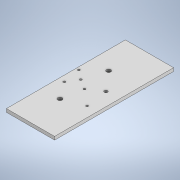
# Autodesk Inventor part: Część1
Saved by Autodesk Inventor 2020 (Build 240168000, 168)
## iProperties
Created: 2019-04-24
Part Number: Część1
Material: Ogólny
Document SubType Name: Modeling
Designer: atmat
Density: 1 g/cm^3
Appearance: Domyślna
Author: atmat
Autodesk Inventor part; units mm, degrees
ref_plane "YZ Plane" through (0, 0, 0) normal (1, 0, 0) x (0, 1, 0)
ref_plane "XZ Plane" through (0, 0, 0) normal (0, 1, 0) x (-1, 0, 0)
ref_plane "XY Plane" through (0, 0, 0) normal (0, 0, 1) x (1, 0, 0)
sketch "Szkic1" plane through (0, 0, 0) normal (0, 1, 0) x (-1, 0, 0)
  circle A0 centre (0, 22.5) radius 2
  circle A1 centre (0, -22.5) radius 2
  circle A2 centre (0, 22.5) radius 11.25 construction
  circle A3 centre (0, -22.5) radius 11.25 construction
  circle A4 centre (0, 0) radius 11.25
  circle A5 centre (-15.3043, -4.6667) radius 4.75 construction
  circle A6 centre (-15.3043, -4.6667) radius 12.25 construction
  circle A7 centre (-18.2464, 15.6211) radius 8.25 construction
  circle A8 centre (-18.2464, 15.6211) radius 1
  circle A9 centre (-15.3043, -4.6667) radius 1.5
  line L0 (17, 55) -> (-27.5543, 55)
  line L1 (-27.5543, 55) -> (-27.5543, -55)
  line L2 (-27.5543, -55) -> (17, -55)
  line L3 (17, -55) -> (17, 55)
  circle A10 centre (0, 22.5) radius 17 construction
  circle A11 centre (0, -22.5) radius 17 construction
  circle A12 centre (0, 0) radius 14.5 construction
  line L4 (12.5, 7.3485) -> (12.5, -7.3485) construction
  line L5 (-12.5, 7.3485) -> (-12.5, -7.3485) construction
  circle A13 centre (14.4557, -9.4125) radius 8.25 construction
  circle A14 centre (14.4557, -9.4125) radius 2.75 construction
  circle A15 centre (11.623, 6.8425) radius 8.25 construction
  circle A16 centre (11.623, 6.8425) radius 1
  circle A17 centre (14.4557, -9.4125) radius 1
  circle A18 centre (5.8715, -2.5341) radius 8.25 construction
  circle A19 centre (5.8715, -2.5341) radius 1
  circle A20 centre (5.8715, -2.5341) radius 2.75 construction
  circle A21 centre (-3.4492, 3.3075) radius 8.25 construction
  circle A22 centre (-3.4492, 3.3075) radius 1
  circle A23 centre (-3.4492, 3.3075) radius 2.75 construction
  dimension "d0" = 4
  dimension "d1" = 4
  dimension "d2" = 22.5
  dimension "d3" = 22.5
  dimension "d4" = 22.5
  dimension "d5" = 22.5
  dimension "d6" = 22.5
  dimension "d7" = 9.5
  dimension "d8" = 24.5
  dimension "d9" = 16.5
  dimension "d10" = 2
  dimension "d11" = 3
  dimension "d12" = 34
  dimension "d13" = 34
  dimension "d14" = 29
  dimension "d15" = 25
  dimension "d16" = 17
  dimension "d17" = 55
  dimension "d18" = 110
  dimension "d21" = 16.5
  dimension "d22" = 5.5
  dimension "d23" = 16.5
  dimension "d24" = 45
  dimension "d26" = 2
  dimension "d27" = 2
  dimension "d28" = 16.5
  dimension "d29" = 2
  dimension "d30" = 5.5
  dimension "d33" = 16.5
  dimension "d34" = 27.5543
  dimension "d35" = 2
  dimension "d36" = 5.5
  constraints: 24 centre point, 16 coincident, 13 tangent, 12 end point, 4 parallel, 4 point on circle, 1 horizontal, 1 perpendicular, 1 vertical
  measures "d0" diameter of A0
  measures "d1" diameter of A1
  measures "d2" distance of point (0, 0) A0.centre
  measures "d3" distance of point (0, 0) A1.centre
  measures "d4" diameter of A2
  measures "d5" diameter of A3
  measures "d6" diameter of A4
  measures "d7" diameter of A5
  measures "d8" diameter of A6
  measures "d9" diameter of A7
  measures "d10" diameter of A8
  measures "d11" diameter of A9
  measures "d12" diameter of A10
  measures "d13" diameter of A11
  measures "d14" diameter of A12
  measures "d15" distance between parallel lines of L4 L5
  measures "d16" distance from line of L3 A4.centre
  measures "d17" distance from line of point (0, 0) L0
  measures "d18" distance between parallel lines of L2 L0
  measures "d21" diameter of A13
  measures "d22" diameter of A14
  measures "d23" diameter of A15
  measures "d24" distance of A0.centre A1.centre
  measures "d26" diameter of A16
  measures "d27" diameter of A17
  measures "d28" diameter of A18
  measures "d29" diameter of A19
  measures "d30" diameter of A20
  measures "d33" diameter of A21
  measures "d34" distance from line of L1 A1.centre
  measures "d35" diameter of A22
  measures "d36" diameter of A23
extrude "Wyciągnięcie proste3" add sketch "Szkic1" along normal blind 3 contours A4 | L3 L2 L1 L0
